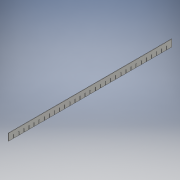
# Autodesk Inventor part: DividerLengthPlastic
Saved by Autodesk Inventor 2016 (Build 200138000, 138)
## iProperties
Created: 2016-02-08
Part Number: DividerLengthPlastic
Material: ABS Plastic
Document SubType Name: Modeling
Designer: ron
Density: 1.06 g/cm^3
Appearance: Smooth - White
Mass: 200.03 g
Surface Area: 1319.35 cm^2
Volume: 188.707 cm^3
Author: ron
Autodesk Inventor part; units mm, degrees
ref_plane "YZ Plane" through (0, 0, 0) normal (1, 0, 0) x (0, 1, 0)
ref_plane "XZ Plane" through (0, 0, 0) normal (0, 1, 0) x (-1, 0, 0)
ref_plane "XY Plane" through (0, 0, 0) normal (0, 0, 1) x (1, 0, 0)
sketch "Sketch1" plane through (0, 0, 0) normal (1, 0, 0) x (0, 1, 0)
  line L0 (0, 0) -> (50.8, 0)
  line L1 (50.8, 0) -> (50.8, -1219.2)
  line L2 (50.8, -1219.2) -> (0, -1219.2)
  line L3 (0, -1219.2) -> (0, -1182.6875)
  line L4 (0, -1182.6875) -> (25.4, -1182.6875)
  line L5 (25.4, -1182.6875) -> (25.4, -1179.5125)
  line L6 (25.4, -1179.5125) -> (0, -1179.5125)
  line L7 (0, -1179.5125) -> (0, -1144.5875)
  line L8 (0, -1144.5875) -> (25.4, -1144.5875)
  line L9 (25.4, -1144.5875) -> (25.4, -1141.4125)
  line L10 (25.4, -1141.4125) -> (0, -1141.4125)
  line L11 (0, -1141.4125) -> (0, -1106.4875)
  line L12 (0, -1106.4875) -> (25.4, -1106.4875)
  line L13 (25.4, -1106.4875) -> (25.4, -1103.3125)
  line L14 (25.4, -1103.3125) -> (0, -1103.3125)
  line L15 (0, -1103.3125) -> (0, -1068.3875)
  line L16 (0, -1068.3875) -> (25.4, -1068.3875)
  line L17 (25.4, -1068.3875) -> (25.4, -1065.2125)
  line L18 (25.4, -1065.2125) -> (0, -1065.2125)
  line L19 (0, -1065.2125) -> (0, -1030.2875)
  line L20 (0, -1030.2875) -> (25.4, -1030.2875)
  line L21 (25.4, -1030.2875) -> (25.4, -1027.1125)
  line L22 (25.4, -1027.1125) -> (0, -1027.1125)
  line L23 (0, -1027.1125) -> (0, -992.1875)
  line L24 (0, -992.1875) -> (25.4, -992.1875)
  line L25 (25.4, -992.1875) -> (25.4, -989.0125)
  line L26 (25.4, -989.0125) -> (0, -989.0125)
  line L27 (0, -989.0125) -> (0, -954.0875)
  line L28 (0, -954.0875) -> (25.4, -954.0875)
  line L29 (25.4, -954.0875) -> (25.4, -950.9125)
  line L30 (25.4, -950.9125) -> (0, -950.9125)
  line L31 (0, -950.9125) -> (0, -915.9875)
  line L32 (0, -915.9875) -> (25.4, -915.9875)
  line L33 (25.4, -915.9875) -> (25.4, -912.8125)
  line L34 (25.4, -912.8125) -> (0, -912.8125)
  line L35 (0, -912.8125) -> (0, -877.8875)
  line L36 (0, -877.8875) -> (25.4, -877.8875)
  line L37 (25.4, -877.8875) -> (25.4, -874.7125)
  line L38 (25.4, -874.7125) -> (0, -874.7125)
  line L39 (0, -874.7125) -> (0, -839.7875)
  line L40 (0, -839.7875) -> (25.4, -839.7875)
  line L41 (25.4, -839.7875) -> (25.4, -836.6125)
  line L42 (25.4, -836.6125) -> (0, -836.6125)
  line L43 (0, -836.6125) -> (0, -801.6875)
  line L44 (0, -801.6875) -> (25.4, -801.6875)
  line L45 (25.4, -801.6875) -> (25.4, -798.5125)
  line L46 (25.4, -798.5125) -> (0, -798.5125)
  line L47 (0, -798.5125) -> (0, -763.5875)
  line L48 (0, -763.5875) -> (25.4, -763.5875)
  line L49 (25.4, -763.5875) -> (25.4, -760.4125)
  line L50 (25.4, -760.4125) -> (0, -760.4125)
  line L51 (0, -760.4125) -> (0, -725.4875)
  line L52 (0, -725.4875) -> (25.4, -725.4875)
  line L53 (25.4, -725.4875) -> (25.4, -722.3125)
  line L54 (25.4, -722.3125) -> (0, -722.3125)
  line L55 (0, -722.3125) -> (0, -687.3875)
  line L56 (0, -687.3875) -> (25.4, -687.3875)
  line L57 (25.4, -687.3875) -> (25.4, -684.2125)
  line L58 (25.4, -684.2125) -> (0, -684.2125)
  line L59 (0, -684.2125) -> (0, -649.2875)
  line L60 (0, -649.2875) -> (25.4, -649.2875)
  line L61 (25.4, -649.2875) -> (25.4, -646.1125)
  line L62 (25.4, -646.1125) -> (0, -646.1125)
  line L63 (0, -646.1125) -> (0, -611.1875)
  line L64 (0, -611.1875) -> (25.4, -611.1875)
  line L65 (25.4, -611.1875) -> (25.4, -608.0125)
  line L66 (25.4, -608.0125) -> (0, -608.0125)
  line L67 (25.4, -573.0875) -> (25.4, -569.9125)
  line L68 (25.4, -531.8125) -> (0, -531.8125)
  line L69 (0, -573.0875) -> (25.4, -573.0875)
  line L70 (25.4, -569.9125) -> (0, -569.9125)
  line L71 (0, -569.9125) -> (0, -534.9875)
  line L72 (0, -534.9875) -> (25.4, -534.9875)
  line L73 (0, -608.0125) -> (0, -573.0875)
  line L74 (25.4, -534.9875) -> (25.4, -531.8125)
  line L75 (25.4, -496.8875) -> (25.4, -493.7125)
  line L76 (25.4, -455.6125) -> (0, -455.6125)
  line L77 (0, -496.8875) -> (25.4, -496.8875)
  line L78 (25.4, -493.7125) -> (0, -493.7125)
  line L79 (0, -493.7125) -> (0, -458.7875)
  line L80 (0, -458.7875) -> (25.4, -458.7875)
  line L81 (0, -531.8125) -> (0, -496.8875)
  line L82 (25.4, -458.7875) -> (25.4, -455.6125)
  line L83 (25.4, -420.6875) -> (25.4, -417.5125)
  line L84 (25.4, -379.4125) -> (0, -379.4125)
  line L85 (0, -420.6875) -> (25.4, -420.6875)
  line L86 (25.4, -417.5125) -> (0, -417.5125)
  line L87 (0, -417.5125) -> (0, -382.5875)
  line L88 (0, -382.5875) -> (25.4, -382.5875)
  line L89 (0, -455.6125) -> (0, -420.6875)
  line L90 (25.4, -382.5875) -> (25.4, -379.4125)
  line L91 (25.4, -344.4875) -> (25.4, -341.3125)
  line L92 (25.4, -303.2125) -> (0, -303.2125)
  line L93 (0, -344.4875) -> (25.4, -344.4875)
  line L94 (25.4, -341.3125) -> (0, -341.3125)
  line L95 (0, -341.3125) -> (0, -306.3875)
  line L96 (0, -306.3875) -> (25.4, -306.3875)
  line L97 (0, -379.4125) -> (0, -344.4875)
  line L98 (25.4, -306.3875) -> (25.4, -303.2125)
  line L99 (25.4, -268.2875) -> (25.4, -265.1125)
  line L100 (25.4, -227.0125) -> (0, -227.0125)
  line L101 (0, -268.2875) -> (25.4, -268.2875)
  line L102 (25.4, -265.1125) -> (0, -265.1125)
  line L103 (0, -265.1125) -> (0, -230.1875)
  line L104 (0, -230.1875) -> (25.4, -230.1875)
  line L105 (0, -303.2125) -> (0, -268.2875)
  line L106 (25.4, -230.1875) -> (25.4, -227.0125)
  line L107 (25.4, -192.0875) -> (25.4, -188.9125)
  line L108 (25.4, -150.8125) -> (0, -150.8125)
  line L109 (0, -192.0875) -> (25.4, -192.0875)
  line L110 (25.4, -188.9125) -> (0, -188.9125)
  line L111 (0, -188.9125) -> (0, -153.9875)
  line L112 (0, -153.9875) -> (25.4, -153.9875)
  line L113 (0, -227.0125) -> (0, -192.0875)
  line L114 (25.4, -153.9875) -> (25.4, -150.8125)
  line L115 (25.4, -115.8875) -> (25.4, -112.7125)
  line L116 (25.4, -74.6125) -> (0, -74.6125)
  line L117 (0, -115.8875) -> (25.4, -115.8875)
  line L118 (25.4, -112.7125) -> (0, -112.7125)
  line L119 (0, -112.7125) -> (0, -77.7875)
  line L120 (0, -77.7875) -> (25.4, -77.7875)
  line L121 (0, -150.8125) -> (0, -115.8875)
  line L122 (25.4, -77.7875) -> (25.4, -74.6125)
  line L123 (25.4, -39.6875) -> (25.4, -36.5125)
  line L124 (25.4, 0) -> (0, 0)
  line L125 (0, -39.6875) -> (25.4, -39.6875)
  line L126 (25.4, -36.5125) -> (0, -36.5125)
  line L127 (0, -36.5125) -> (0, 0)
  line L128 (0, -74.6125) -> (0, -39.6875)
  dimension "d364" = 50.8
  dimension "d365" = 1219.2
  dimension "d377" = 36.5125
  dimension "d379" = 25.4
  dimension "d380" = 3.175
  dimension "d381" = 34.925
  dimension "d382" = 25.4
  dimension "d383" = 3.175
  dimension "d384" = 34.925
  dimension "d385" = 25.4
  dimension "d386" = 3.175
  dimension "d387" = 34.925
  dimension "d388" = 25.4
  dimension "d389" = 3.175
  dimension "d390" = 34.925
  dimension "d391" = 25.4
  dimension "d392" = 3.175
  dimension "d393" = 34.925
  dimension "d394" = 25.4
  dimension "d395" = 3.175
  dimension "d396" = 34.925
  dimension "d397" = 25.4
  dimension "d398" = 3.175
  dimension "d399" = 34.925
  dimension "d400" = 25.4
  dimension "d401" = 3.175
  dimension "d402" = 34.925
  dimension "d403" = 25.4
  dimension "d404" = 3.175
  dimension "d405" = 34.925
  dimension "d406" = 25.4
  dimension "d407" = 3.175
  dimension "d408" = 34.925
  dimension "d409" = 25.4
  dimension "d410" = 3.175
  dimension "d411" = 34.925
  dimension "d412" = 25.4
  dimension "d413" = 3.175
  dimension "d414" = 34.925
  dimension "d415" = 25.4
  dimension "d416" = 3.175
  dimension "d417" = 34.925
  dimension "d418" = 25.4
  dimension "d419" = 3.175
  dimension "d420" = 34.925
  dimension "d421" = 25.4
  dimension "d422" = 3.175
  dimension "d423" = 34.925
  dimension "d424" = 25.4
  dimension "d425" = 3.175
  dimension "d426" = 34.925
  dimension "d427" = 25.4
  dimension "d428" = 3.175
  dimension "d429" = 34.925
  dimension "d430" = 25.4
  dimension "d431" = 3.175
  dimension "d432" = 34.925
  dimension "d433" = 25.4
  dimension "d434" = 3.175
  dimension "d435" = 34.925
  dimension "d436" = 25.4
  dimension "d437" = 3.175
  dimension "d438" = 34.925
  dimension "d439" = 25.4
  constraints: 259 end point, 65 perpendicular, 46 point on line, 17 horizontal, 16 vertical, 15 parallel, 1 midpoint
  measures "d364" distance of L0.start L0.end
  measures "d365" distance of L0.end L1.end
  measures "d377" distance of L2.end L3.end
  measures "d379" distance of L3.end L4.end
  measures "d380" distance of L4.end L5.end
  measures "d381" distance of L6.end L7.end
  measures "d382" distance of L7.end L8.end
  measures "d383" distance of L8.end L9.end
  measures "d384" distance of L10.end L12.start
  measures "d385" distance of L12.start L13.start
  measures "d386" distance of L13.start L13.end
  measures "d387" distance of L14.end L15.end
  measures "d388" distance of L15.end L16.end
  measures "d389" distance of L16.end L18.start
  measures "d390" distance of L18.end L20.start
  measures "d391" distance of L20.start L21.start
  measures "d392" distance of L21.start L21.end
  measures "d393" distance of L22.end L23.end
  measures "d394" distance of L23.end L24.end
  measures "d395" distance of L24.end L26.start
  measures "d396" distance of L26.end L28.start
  measures "d397" distance of L28.start L29.start
  measures "d398" distance of L29.start L29.end
  measures "d399" distance of L30.end L31.end
  measures "d400" distance of L31.end L32.end
  measures "d401" distance of L32.end L34.start
  measures "d402" distance of L34.end L36.start
  measures "d403" distance of L36.start L37.start
  measures "d404" distance of L37.start L37.end
  measures "d405" distance of L38.end L39.end
  measures "d406" distance of L39.end L40.end
  measures "d407" distance of L40.end L42.start
  measures "d408" distance of L42.end L44.start
  measures "d409" distance of L44.start L45.start
  measures "d410" distance of L45.start L45.end
  measures "d411" distance of L46.end L47.end
  measures "d412" distance of L47.end L48.end
  measures "d413" distance of L48.end L50.start
  measures "d414" distance of L50.end L52.start
  measures "d415" distance of L52.start L53.start
  measures "d416" distance of L53.start L53.end
  measures "d417" distance of L54.end L55.end
  measures "d418" distance of L55.end L56.end
  measures "d419" distance of L56.end L58.start
  measures "d420" distance of L58.end L60.start
  measures "d421" distance of L60.start L61.start
  measures "d422" distance of L61.start L61.end
  measures "d423" distance of L62.end L63.end
  measures "d424" distance of L63.end L64.end
  measures "d425" distance of L64.end L66.start
  measures "d426" distance of L66.end L73.end
  measures "d427" distance of L73.end L67.start
  measures "d428" distance of L67.start L70.start
  measures "d429" distance of L70.end L72.start
  measures "d430" distance of L72.start L72.end
  measures "d431" distance of L72.end L68.start
  measures "d432" distance of L68.end L81.end
  measures "d433" distance of L81.end L77.end
  measures "d434" distance of L77.end L75.end
  measures "d435" distance of L78.end L79.end
  measures "d436" distance of L79.end L82.start
  measures "d437" distance of L82.start L76.start
  measures "d438" distance of L76.end L89.end
  measures "d439" distance of L89.end L83.start
extrude "Extrusion2" add sketch "Sketch1" along normal blind 3.175
body "Solid2"
